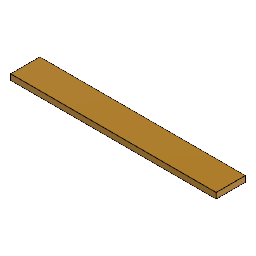
tube_holder_210806_2x8 v59 (Autodesk Fusion 360 archive; units mm, degrees)
design "HeatRubber"
Autodesk Fusion 360 part; units mm, degrees
box "BoxPrimitive1" add length 10 width 80 height 2 placed x (0, 1, 0) y (-1, 0, 0) z (0, 0, 1) at (80, 0, 0)
move_body "Move1" bodies 1 to x (1, 0, 0) y (0, 1, 0) z (0, 0, 1) at (-40, -5, 0)
extrude "Extrude1" cut 1 faces at (40, -1.6667, 0.6667) along direction (-1, 0, 0) blind 5
extrude "Extrude2" cut 1 faces at (-40, -1.6667, 0.6667) along direction (1, 0, 0) blind 5

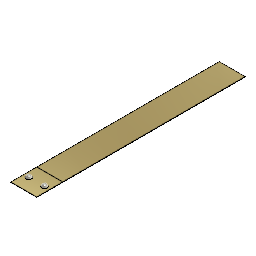
design "well_heater"
Autodesk Fusion 360 part; units mm, degrees
box "BoxPrimitive1" add length 80 width 10 height 0.2 placed x (0, 1, 0) y (-1, 0, 0) z (0, 0, 1) at (10, 0, 0) makes body 1
extrude "Extrude1" add 1 faces at (3.3333, 0, 0.0667) along direction (0, 1, 0) blind 10 separate body on bodies 1 makes body 2
sketch "Sketch2" plane through (0, 0, 0.2) normal (0, 0, 1) x (-1, 0, 0)
  line L0 (0, 0) -> (-10, 0)
  line L1 (-10, 0) -> (-10, -10)
  line L2 (-10, -10) -> (0, -10)
  line L3 (0, -10) -> (0, 0)
  line L4 (-2, -5) -> (-8, -5)
  line L5 (-8, -5) -> (-8, -15)
  line L6 (-8, -15) -> (-2, -15)
  line L7 (-2, -15) -> (-2, -5)
  line L8 (-2, -5) -> (-8, -15) construction
  line L9 (-8, -5) -> (-2, -15) construction
  circle A0 centre (-2, -5) radius 1
  circle A1 centre (-8, -5) radius 1
  point P0 (-5, -10)
  dimension "d1" = 6
  dimension "d2" = 10
  dimension "d3" = 2
  dimension "d4" = 2
  constraint horizontal L4
  constraint perpendicular L4 L5
  constraint parallel L4 L6
  constraint parallel L5 L7
  constraint coincident L8 P0
  constraint coincident L9 P0
  constraint midpoint L2 P0
  constraint coincident L4.start L7.end
  constraint coincident L4.end L5.start
  measures "d1" distance of L5.end L6.end
  measures "d2" distance of L4.end L5.end
  measures "d3" diameter of A0
  measures "d4" diameter of A1
extrude "Extrude2" add sketch "Sketch2" along normal blind 1 separate body contours L4 L7 A0 | L4 L7 A0 | L4 L5 A1 | L4 L5 A1 makes body 3 at (7.005, 5.0996, 0.5333) makes body 4 at (1.005, 5.0996, 0.5333)
copy_body "Body->Comp1" bodies 3 removing the originals makes body 5 in component "tab1"
copy_body "Body->Comp2" bodies 4 removing the originals makes body 6 in component "tab2"
fillet "Fillet1" radius 1 1 edges at (2.9323, 5.3616, 1.2) on bodies 6 in component "tab2"
fillet "Fillet1'" radius 1 1 edges at (8.9323, 5.3616, 1.2) on bodies 5 in component "tab1"
component "tab1" placed x (1, 0, 0) y (0, 1, 0) z (0, 0, 1) at (0, 0, 0)
component "tab2" placed x (1, 0, 0) y (0, 1, 0) z (0, 0, 1) at (0, 0, 0)
